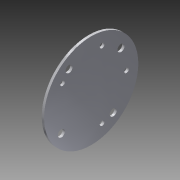
# Autodesk Inventor part: plate
Saved by Autodesk Inventor 2015 (Build 190159000, 159)
## iProperties
Created: 2015-12-22
Part Number: plate
Material: アルミニウム 6061
Document SubType Name: Modeling
Designer: Ryo
Density: 2.7 g/cm^3
Appearance: アルミニウム - フラット
Author: Ryo
Autodesk Inventor part; units mm, degrees
ref_plane "YZ Plane" through (0, 0, 0) normal (1, 0, 0) x (0, 1, 0)
ref_plane "XZ Plane" through (0, 0, 0) normal (0, 1, 0) x (-1, 0, 0)
ref_plane "XY Plane" through (0, 0, 0) normal (0, 0, 1) x (1, 0, 0)
sketch "スケッチ1" plane through (0, 0, 0) normal (1, 0, 0) x (0, 1, 0)
  circle A0 centre (0, 0) radius 40
  circle A1 centre (30, 0) radius 2
  circle A2 centre (9.2705, 28.5317) radius 2
  circle A3 centre (-24.2705, 17.6336) radius 2
  circle A4 centre (-24.2705, -17.6336) radius 2
  circle A5 centre (9.2705, -28.5317) radius 2
  circle A6 centre (0, 0) radius 31.5
  circle A7 centre (-25.3153, -18.7453) radius 3
  circle A8 centre (18.7453, -25.3153) radius 3
  circle A9 centre (25.3153, 18.7453) radius 3
  circle A10 centre (-18.7453, 25.3153) radius 3
  dimension "d0" = 80
  dimension "d1" = 30
  dimension "d2" = 4
  dimension "d5" = 360
  dimension "d7" = 63
  dimension "d8" = 6
  dimension "d11" = 360
  constraints: 11 centre point, 2 coincident, 20 other
  measures "d0" diameter of A0
  measures "d1" distance of point (0, 0) A1.centre
  measures "d2" diameter of A1
  measures "d7" diameter of A6
  measures "d8" diameter of A7
extrude "押し出し1" add sketch "スケッチ1" along normal blind 2 contours A0 | A1 A6 | A6 A1 | A1 A6 A8 A5 A7 A4 A3 A10 A2 A9 | A9 A6 | A6 A9 | A8 A6 | A6 A8 | A6 A2 | A2 A6 | A6 A5 | A5 A6 | A10 A6 | A6 A10 | A7 A6 A4 | A6 A4 A7 | A6 A4 A7 | A4 A6 | A7 A4 A6 | A6 A3 | A3 A6 | A7 A4
extrude "押し出し2" cut sketch "スケッチ1" along normal blind 2 contours A1 A6 | A6 A1 | A9 A6 | A6 A9 | A8 A6 | A6 A8 | A6 A2 | A2 A6 | A6 A5 | A5 A6 | A10 A6 | A6 A10 | A7 A6 A4 | A6 A4 A7 | A6 A4 A7 | A4 A6 | A7 A4 A6 | A6 A3 | A3 A6
